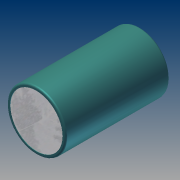
# Autodesk Inventor part: D Cell
Saved by Autodesk Inventor 2012 SP1 (Build 160190100, 190)
## iProperties
Created: 2011-12-06
Part Number: D Cell
Material: Default
Document SubType Name: Modeling
Designer: Jon
Density: 1.88883 g/cm^3
Mass: 100 g
Surface Area: 84.7834 cm^2
Volume: 52.9428 cm^3
Author: Jon
Autodesk Inventor part; units mm, degrees
ref_plane "YZ Plane" through (0, 0, 0) normal (1, 0, 0) x (0, 1, 0)
ref_plane "XZ Plane" through (0, 0, 0) normal (0, 1, 0) x (-1, 0, 0)
ref_plane "XY Plane" through (0, 0, 0) normal (0, 0, 1) x (1, 0, 0)
sketch "Sketch1" plane through (0, 0, 0) normal (0, 0, 1) x (1, 0, 0)
  line L0 (-16.8, -30.65) -> (0, -30.65)
  line L1 (0, -30.65) -> (0, 30.65)
  line L2 (0, 30.65) -> (-16.8, 30.65)
  line L3 (-16.8, 30.65) -> (-16.8, -30.65)
  point P0 (0, 0)
  point P1 (0, 0)
  dimension "d0" = 16.8
  dimension "d1" = 61.3
  constraints: 8 end point, 2 parallel, 1 coincident, 1 horizontal, 1 midpoint, 1 perpendicular
  measures "d0" distance of L2.end L1.end
  measures "d1" distance of L1.end L0.end
revolve "Revolution1" add sketch "Sketch1" angle 360 about axis through (0, -30.65, 0) along (0, 1, 0)
sketch "Sketch2" plane through (0, 30.65, 0) normal (0, 1, 0) x (1, 0, 0)
  circle A0 centre (0, 0) radius 16.8 projected
  circle A1 centre (0, 0) radius 12.5
  circle A2 centre (0, 0) radius 5
  dimension "d3" = 10
  dimension "d4" = 7.5
  constraints: 2 centre point
  measures "d3" diameter of A2
  measures "d4" radial gap between concentric circles of A2 A1
extrude "Extrusion1" cut sketch "Sketch2" against normal blind 5 contours A1
sketch "Sketch3" plane through (0, 30.65, 0) normal (0, 1, 0) x (1, 0, 0)
  circle A0 centre (0, 0) radius 16.8 projected
  circle A1 centre (0, 0) radius 12.5 projected
extrude "Extrusion2" cut sketch "Sketch3" against normal blind 2
fillet "Fillet1" radius 1 3 edges at (16.8, -30.65, 0) (16.8, 28.65, 0) (-12.5, 28.65, 0)
sketch "Sketch4" plane through (0, 30.65, 0) normal (0, 1, 0) x (1, 0, 0)
  circle A0 centre (0, 0) radius 5 projected
  circle A1 centre (0, 0) radius 4
  dimension "d10" = 1
  constraints: 1 centre point
  measures "d10" radial gap between concentric circles of A1 A0
extrude "Extrusion3" cut sketch "Sketch4" against normal blind 2
chamfer "Chamfer1" distance 2 angle 45 1 edges at (-5, 25.65, 0)
sketch "Sketch5" plane through (0, -30.65, 0) normal (0, -1, 0) x (1, 0, 0)
  circle A0 centre (0, 0) radius 15.8 projected
  circle A1 centre (0, 0) radius 15
  dimension "d16" = 30
  constraints: 1 centre point
  measures "d16" diameter of A1
extrude "Extrusion4" cut sketch "Sketch5" against normal blind 0.25 contours A1
body "Solid1"
